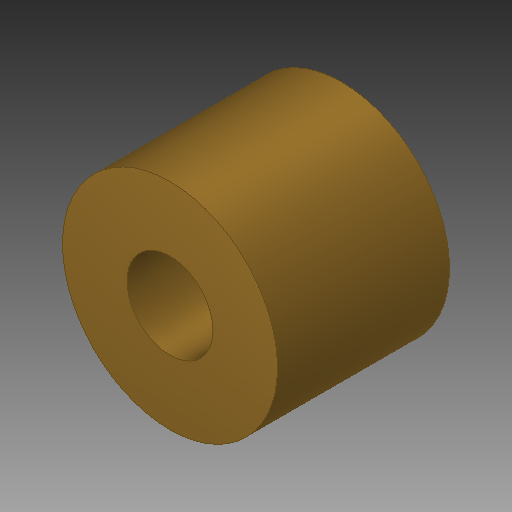
# Autodesk Inventor part: Peça3
Saved by Autodesk Inventor 2018 (Build 220112000, 112)
## iProperties
Created: 2018-05-16
Part Number: Peça3
Material: Latão, amarelo macio
Document SubType Name: Modeling
Designer: Usuario
Density: 8.47 g/cm^3
Appearance: Latão - Acetinado
Author: Usuario
Autodesk Inventor part; units mm, degrees
ref_plane "YZ Plane" through (0, 0, 0) normal (1, 0, 0) x (0, 1, 0)
ref_plane "XZ Plane" through (0, 0, 0) normal (0, 1, 0) x (-1, 0, 0)
ref_plane "XY Plane" through (0, 0, 0) normal (0, 0, 1) x (1, 0, 0)
sketch "Esboço1" plane through (0, 0, 0) normal (0, 0, 1) x (1, 0, 0)
  circle A0 centre (116.7963, 191.7963) radius 2 construction
  line L0 (122, -197) -> (122, 197) construction
  line L1 (122, 197) -> (-122, 197) construction
  circle A1 centre (116.7963, 191.7963) radius 2
  circle A2 centre (116.7963, 191.7963) radius 5
  point P0 (0, 0)
  dimension "d0" = 10
  constraints: 2 centre point, 2 coincident, 1 concentric
  measures "d0" diameter of A2
extrude "Extrusão1" add sketch "Esboço1" along normal blind 8
